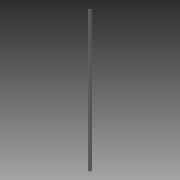
# Autodesk Inventor part: Pied
Saved by Autodesk Inventor 2015 SP1 (Build 190203100, 203)
## iProperties
Created: 2015-04-25
Part Number: Pied
Material: Générique
Document SubType Name: Modeling
Designer: Cyril
Density: 1 g/cm^3
Appearance: Par défaut
Author: Cyril
Autodesk Inventor part; units mm, degrees
ref_plane "YZ Plane" through (0, 0, 0) normal (1, 0, 0) x (0, 1, 0)
ref_plane "XZ Plane" through (0, 0, 0) normal (0, 1, 0) x (-1, 0, 0)
ref_plane "XY Plane" through (0, 0, 0) normal (0, 0, 1) x (1, 0, 0)
sketch "Sketch1" plane through (0, 0, 0) normal (0, 0, 1) x (1, 0, 0)
  line L0 (-12.5, -12.5) -> (12.5, -12.5)
  line L1 (12.5, -12.5) -> (12.5, 12.5)
  line L2 (12.5, 12.5) -> (-12.5, 12.5)
  line L3 (-12.5, 12.5) -> (-12.5, -12.5)
  line L4 (-12.5, -12.5) -> (12.5, 12.5) construction
  line L5 (12.5, -12.5) -> (-12.5, 12.5) construction
  line L6 (-11.5, -11.5) -> (11.5, -11.5)
  line L7 (11.5, -11.5) -> (11.5, 11.5)
  line L8 (11.5, 11.5) -> (-11.5, 11.5)
  line L9 (-11.5, 11.5) -> (-11.5, -11.5)
  line L10 (-11.5, -11.5) -> (11.5, 11.5) construction
  line L11 (11.5, -11.5) -> (-11.5, 11.5) construction
  point P0 (0, 0)
  dimension "d0" = 25
  dimension "d1" = 25
  dimension "d2" = 1
  constraints: 24 end point, 4 midpoint, 4 parallel, 2 horizontal, 2 perpendicular, 1 point on line
  measures "d0" distance of L1.end L2.end
  measures "d1" distance of L2.end L0.start
  measures "d2" distance between parallel lines of L2 L8
extrude "Extrusion1" add sketch "Sketch1" along normal mid plane 1678
sketch "Sketch2" plane through (12.5, -12.5, 839) normal (1, 0, 0) x (0, 0, -1)
  circle A0 centre (1658, 12.5) radius 10
  line L0 (1678, 25) -> (1678, 0) projected
  line L1 (1658, 12.5) -> (1678, 12.5) construction
  point P0 (839, 12.5)
  dimension "d5" = 20
  dimension "d6" = 20
  constraints: 2 end point, 1 centre point, 1 midpoint, 1 perpendicular
  measures "d5" diameter of A0
  measures "d6" distance from line of L0 L1.start
extrude "Extrusion2" cut sketch "Sketch2" against normal through all
sketch "Sketch3" plane through (12.5, -12.5, 839) normal (1, 0, 0) x (0, 0, -1)
  line L0 (0, 0) -> (8.123, 25)
  line L1 (8.123, 25) -> (0, 25)
  line L2 (0, 25) -> (0, 0)
  line L3 (1678, 25) -> (0, 25) projected
  point P0 (839, 12.5)
  dimension "d9" = 18
  constraints: 6 end point, 1 coincident, 1 horizontal, 1 perpendicular, 1 point on line
  measures "d9" angle of L2 L0
extrude "Extrusion3" cut sketch "Sketch3" against normal through all
body "Solid1"
